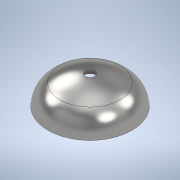
# Autodesk Inventor part: ODSY-0004-002
Saved by Autodesk Inventor 2021 (Build 250183000, 183)
## iProperties
Created: 2021-08-03
Part Number: ODSY-0004-002
Material: Stainless Steel, 440C
Document SubType Name: Modeling
Designer: ALEX CLAY
Density: 7.75 g/cm^3
Appearance: Semi-Polished
Mass: 9130.58 g
Surface Area: 2575.45 cm^2
Volume: 1178.14 cm^3
Project: ODYSSEY
Description: Tank Cap
Author: Alex Clay
Title: Tank Cap
Revision Number: 0
Autodesk Inventor part; units mm, degrees
ref_plane "YZ Plane" through (0, 0, 0) normal (1, 0, 0) x (0, 1, 0)
ref_plane "XZ Plane" through (0, 0, 0) normal (0, 1, 0) x (-1, 0, 0)
ref_plane "XY Plane" through (0, 0, 0) normal (0, 0, 1) x (1, 0, 0)
sketch "Sketch1" plane through (0, 0, 0) normal (0, 0, 1) x (1, 0, 0)
  arc A0 (152.4, 0) -> (111.0074, 70.3431) centre (71.9328, 0) ccw
  arc A1 (111.0074, 70.3431) -> (0, 99.1048) centre (0, -129.4952) ccw
  line L0 (152.4, -5.7873) -> (152.4, 0) construction
  line L1 (161.925, 0) -> (161.925, -5.7873) construction
  line L2 (152.4, 0) -> (161.925, 0)
  line L3 (0, 0) -> (0, 14.6977) construction
  arc A2 (161.925, 0) -> (115.6327, 78.6696) centre (71.9328, 0) ccw
  arc A3 (115.6327, 78.6696) -> (0, 108.6298) centre (0, -129.4952) ccw
  line L4 (0, 99.1048) -> (0, 108.6298)
  dimension "d1" = 9.525
  dimension "d2" = 161.925
  dimension "d3" = 228.6
  dimension "d4" = 80.4672
  constraints: 10 end point, 8 point on circle, 4 centre point, 4 vertical, 3 tangent, 2 coincident, 2 horizontal alignment, 2 vertical alignment, 1 horizontal, 1 point on line
  measures "d1" distance between parallel lines of L1 L0
  measures "d2" distance between parallel lines of L1 L3
  measures "d3" radius of A1
  measures "d4" radius of A0
revolve "Revolution1" add sketch "Sketch1" angle 360 about axis through (0, 0, 0) along (0, 1, 0)
sketch "Sketch2" plane through (0, 0, 0) normal (0, -1, 0) x (1, 0, 0)
  circle A0 centre (0, 0) radius 17.4625
  dimension "d6" = 34.925
  constraints: 1 centre point, 1 coincident
  measures "d6" diameter of A0
extrude "Extrusion1" cut sketch "Sketch2" against normal through all
equation "\"d3\" = -1.5 * d1 + 1.5 * d2"
equation "\"d4\" = -0.528 * d1 + 0.528 * d2"
body "Solid1"
